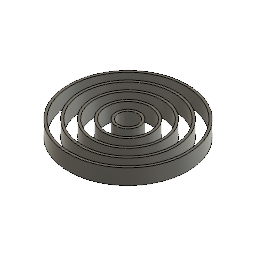
3Dprinting rings (Autodesk Fusion 360 design; units mm, degrees)
Autodesk Fusion 360 part; units mm, degrees
sketch "Sketch1" plane through (0, 0, 0) normal (0, 1, 0) x (1, 0, 0)
  circle A0 centre (15, -5) radius 50
  circle A1 centre (15, -5) radius 48
  circle A2 centre (15, -5) radius 40
  circle A3 centre (15, -5) radius 38
  circle A4 centre (15, -5) radius 30
  circle A5 centre (15, -5) radius 28
  circle A6 centre (15, -5) radius 20
  circle A7 centre (15, -5) radius 18
  circle A8 centre (15, -5) radius 10
  circle A9 centre (15, -5) radius 8
  dimension "d2" = -2
  dimension "d4" = -2
  dimension "d6" = -2
  dimension "d8" = -2
  dimension "d10" = -2
extrude "Extrude1" add sketch "Sketch1" along normal blind 13 makes body 1 at (44.8509, 8.6667, 7.987) makes body 2 at (54.8012, 8.6667, 8.9827) makes body 3 at (34.9006, 8.6667, 6.9914) makes body 4 at (64.7515, 8.6667, 9.9784) makes body 5 at (24.9503, 8.6667, 5.9957)
